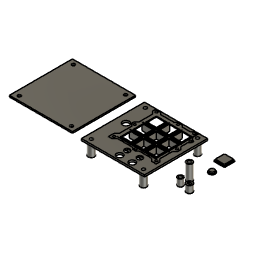
tic_tac_toe (Autodesk Fusion 360 design; units mm, degrees)
Autodesk Fusion 360 part; units mm, degrees
sketch "Sketch1" plane through (0, 0, 0) normal (0, 0, 1) x (1, 0, 0)
  line L0 (0, 0) -> (70, 0)
  line L1 (70, 0) -> (70, 70)
  line L2 (70, 70) -> (0, 70)
  line L3 (0, 70) -> (0, 0)
  circle A0 centre (6, 65) radius 1.75
  circle A1 centre (64, 65) radius 1.75
  circle A2 centre (64, 5) radius 1.75
  circle A3 centre (6, 5) radius 1.75
  line L4 (19, 64.2) -> (32, 64.2)
  line L5 (32, 64.2) -> (32, 51.2)
  line L6 (32, 51.2) -> (19, 51.2)
  line L7 (19, 51.2) -> (19, 64.2)
  line L8 (20, 63.2) -> (31, 63.2)
  line L9 (31, 63.2) -> (31, 52.2)
  line L10 (31, 52.2) -> (20, 52.2)
  line L11 (20, 52.2) -> (20, 63.2)
  line L12 (34, 63.2) -> (45, 63.2)
  line L13 (45, 52.2) -> (34, 52.2)
  line L14 (46, 64.2) -> (46, 51.2)
  line L15 (34, 52.2) -> (34, 63.2)
  line L16 (33, 51.2) -> (33, 64.2)
  line L17 (46, 51.2) -> (33, 51.2)
  line L18 (45, 63.2) -> (45, 52.2)
  line L19 (33, 64.2) -> (46, 64.2)
  line L20 (48, 63.2) -> (59, 63.2)
  line L21 (48, 52.2) -> (48, 63.2)
  line L22 (59, 52.2) -> (48, 52.2)
  line L23 (47, 51.2) -> (47, 64.2)
  line L24 (60, 51.2) -> (47, 51.2)
  line L25 (47, 64.2) -> (60, 64.2)
  line L26 (60, 64.2) -> (60, 51.2)
  line L27 (59, 63.2) -> (59, 52.2)
  line L28 (46, 50.2) -> (46, 37.2)
  line L29 (31, 49.2) -> (31, 38.2)
  line L30 (33, 50.2) -> (46, 50.2)
  line L31 (31, 38.2) -> (20, 38.2)
  line L32 (59, 49.2) -> (59, 38.2)
  line L33 (45, 38.2) -> (34, 38.2)
  line L34 (32, 50.2) -> (32, 37.2)
  line L35 (60, 50.2) -> (60, 37.2)
  line L36 (34, 49.2) -> (45, 49.2)
  line L37 (48, 38.2) -> (48, 49.2)
  line L38 (60, 37.2) -> (47, 37.2)
  line L39 (20, 38.2) -> (20, 49.2)
  line L40 (19, 50.2) -> (32, 50.2)
  line L41 (34, 38.2) -> (34, 49.2)
  line L42 (33, 37.2) -> (33, 50.2)
  line L43 (19, 37.2) -> (19, 50.2)
  line L44 (46, 37.2) -> (33, 37.2)
  line L45 (45, 49.2) -> (45, 38.2)
  line L46 (47, 37.2) -> (47, 50.2)
  line L47 (20, 49.2) -> (31, 49.2)
  line L48 (48, 49.2) -> (59, 49.2)
  line L49 (47, 50.2) -> (60, 50.2)
  line L50 (59, 38.2) -> (48, 38.2)
  line L51 (32, 37.2) -> (19, 37.2)
  line L52 (32, 36.2) -> (32, 23.2)
  line L53 (19, 23.2) -> (19, 36.2)
  line L54 (34, 24.2) -> (34, 35.2)
  line L55 (48, 35.2) -> (59, 35.2)
  line L56 (60, 36.2) -> (60, 23.2)
  line L57 (34, 35.2) -> (45, 35.2)
  line L58 (45, 24.2) -> (34, 24.2)
  line L59 (48, 24.2) -> (48, 35.2)
  line L60 (46, 23.2) -> (33, 23.2)
  line L61 (47, 36.2) -> (60, 36.2)
  line L62 (33, 36.2) -> (46, 36.2)
  line L63 (20, 24.2) -> (20, 35.2)
  line L64 (31, 24.2) -> (20, 24.2)
  line L65 (31, 35.2) -> (31, 24.2)
  line L66 (47, 23.2) -> (47, 36.2)
  line L67 (60, 23.2) -> (47, 23.2)
  line L68 (33, 23.2) -> (33, 36.2)
  line L69 (19, 36.2) -> (32, 36.2)
  line L70 (45, 35.2) -> (45, 24.2)
  line L71 (59, 35.2) -> (59, 24.2)
  line L72 (46, 36.2) -> (46, 23.2)
  line L73 (59, 24.2) -> (48, 24.2)
  line L74 (20, 35.2) -> (31, 35.2)
  line L75 (32, 23.2) -> (19, 23.2)
  circle A4 centre (10, 39.5) radius 3.75
  circle A5 centre (36.9, 14) radius 3
  circle A6 centre (50.9, 14) radius 3
  circle A7 centre (36.9, 14) radius 4
  circle A8 centre (50.9, 14) radius 4
  circle A9 centre (37.25, 5.25) radius 3.5
  circle A10 centre (51.25, 5.25) radius 3.5
  circle A11 centre (16, 67.2) radius 1
  circle A12 centre (58, 67.2) radius 1
  circle A13 centre (16, 43.2) radius 1
  circle A14 centre (16, 20.2) radius 1
  circle A15 centre (63, 20.2) radius 1
  circle A16 centre (63, 43.2) radius 1
  circle A17 centre (40, 20.2) radius 1
  circle A18 centre (40, 67.2) radius 1
  circle A19 centre (63, 58.2) radius 1
  dimension "d1" = 70
  dimension "d2" = 70
  dimension "d3" = 3.5
  dimension "d4" = 6
  dimension "d5" = 5
  dimension "d6" = 3.5
  dimension "d7" = 3.5
  dimension "d8" = 3.5
  dimension "d9" = 6
  dimension "d10" = 5
  dimension "d11" = 6
  dimension "d12" = 5
  dimension "d13" = 5
  dimension "d14" = 6
  dimension "d15" = 13
  dimension "d16" = 13
  dimension "d17" = 19
  dimension "d18" = 5.8
  dimension "d19" = 11
  dimension "d20" = 11
  dimension "d21" = 1
  dimension "d22" = 1
  dimension "d23" = 13
  dimension "d24" = 13
  dimension "d25" = 11
  dimension "d26" = 11
  dimension "d27" = 1
  dimension "d28" = 1
  dimension "d29" = 13
  dimension "d30" = 13
  dimension "d31" = 11
  dimension "d32" = 11
  dimension "d33" = 1
  dimension "d34" = 1
  dimension "d35" = 13
  dimension "d36" = 13
  dimension "d37" = 11
  dimension "d38" = 11
  dimension "d39" = 1
  dimension "d40" = 1
  dimension "d41" = 13
  dimension "d42" = 13
  dimension "d43" = 11
  dimension "d44" = 11
  dimension "d45" = 1
  dimension "d46" = 1
  dimension "d47" = 13
  dimension "d48" = 13
  dimension "d49" = 11
  dimension "d50" = 11
  dimension "d51" = 1
  dimension "d52" = 1
  dimension "d53" = 13
  dimension "d54" = 13
  dimension "d55" = 11
  dimension "d56" = 11
  dimension "d57" = 1
  dimension "d58" = 1
  dimension "d59" = 13
  dimension "d60" = 13
  dimension "d61" = 11
  dimension "d62" = 11
  dimension "d63" = 1
  dimension "d64" = 1
  dimension "d65" = 13
  dimension "d66" = 13
  dimension "d67" = 11
  dimension "d68" = 11
  dimension "d69" = 1
  dimension "d70" = 1
  dimension "d71" = 7.5
  dimension "d72" = 30.5
  dimension "d73" = 10
  dimension "d74" = 6
  dimension "d75" = 14
  dimension "d76" = 36.9
  dimension "d77" = 6
  dimension "d78" = 14
  dimension "d79" = 14
  dimension "d80" = 8
  dimension "d81" = 8
  dimension "d82" = 7
  dimension "d83" = 5.25
  dimension "d84" = 37.25
  dimension "d85" = 7
  dimension "d86" = 14
  dimension "d87" = 5.25
  dimension "d88" = 2
  dimension "d89" = 3
  dimension "d90" = 3
  dimension "d91" = 2
  dimension "d93" = 3
  dimension "d94" = 2
  dimension "d95" = 2
  dimension "d96" = 21
  dimension "d97" = 3
  dimension "d98" = 2
  dimension "d99" = 3
  dimension "d100" = 3
  dimension "d101" = 2
  dimension "d102" = 3
  dimension "d103" = 3
  dimension "d104" = 2
  dimension "d105" = 3
  dimension "d106" = 21
  dimension "d107" = 2
  dimension "d108" = 21
  dimension "d109" = 3
  dimension "d110" = 2
  dimension "d111" = 3
  dimension "d112" = 21
  dimension "d148" = 2
  constraint horizontal L0
  constraint vertical L1
  constraint horizontal L2
  constraint vertical L3
  constraint coincident L0.start L3.end
  constraint horizontal L4
  constraint vertical L5
  constraint horizontal L6
  constraint vertical L7
  constraint horizontal L8
  constraint vertical L9
  constraint horizontal L10
  constraint vertical L11
  constraint horizontal L19
  constraint vertical L14
  constraint horizontal L17
  constraint vertical L16
  constraint horizontal L12
  constraint vertical L18
  constraint horizontal L13
  constraint vertical L15
  constraint horizontal L25
  constraint vertical L26
  constraint horizontal L24
  constraint vertical L23
  constraint horizontal L20
  constraint vertical L27
  constraint horizontal L22
  constraint vertical L21
  constraint horizontal L40
  constraint vertical L34
  constraint horizontal L51
  constraint vertical L43
  constraint horizontal L47
  constraint vertical L29
  constraint horizontal L31
  constraint vertical L39
  constraint horizontal L30
  constraint vertical L28
  constraint horizontal L44
  constraint vertical L42
  constraint horizontal L36
  constraint vertical L45
  constraint horizontal L33
  constraint vertical L41
  constraint horizontal L49
  constraint vertical L35
  constraint horizontal L38
  constraint vertical L46
  constraint horizontal L48
  constraint vertical L32
  constraint horizontal L50
  constraint vertical L37
  constraint horizontal L69
  constraint vertical L52
  constraint horizontal L75
  constraint vertical L53
  constraint horizontal L74
  constraint vertical L65
  constraint horizontal L64
  constraint vertical L63
  constraint horizontal L62
  constraint vertical L72
  constraint horizontal L60
  constraint vertical L68
  constraint horizontal L57
  constraint vertical L70
  constraint horizontal L58
  constraint vertical L54
  constraint horizontal L61
  constraint vertical L56
  constraint horizontal L67
  constraint vertical L66
  constraint horizontal L55
  constraint vertical L71
  constraint horizontal L73
  constraint vertical L59
  constraint concentric A5 A7
  constraint concentric A6 A8
  measures "d1" distance of L0.start L0.end
  measures "d2" distance of L0.start L2.end
  measures "d3" diameter of A0
  measures "d4" distance of L3 A0.centre
  measures "d5" distance of L2 A0.centre
  measures "d6" diameter of A1
  measures "d7" diameter of A2
  measures "d8" diameter of A3
  measures "d9" distance of L1 A1.centre
  measures "d10" distance of L2 A1.centre
  measures "d11" distance of L1 A2.centre
  measures "d12" distance of L0 A2.centre
  measures "d13" distance of L0 A3.centre
  measures "d14" distance of L3 A3.centre
  measures "d15" distance of L4.start L4.end
  measures "d16" distance of L4.start L6.end
  measures "d17" distance of L3 L4.start
  measures "d18" distance of L2 L4
  measures "d19" distance of L8.start L8.end
  measures "d20" distance of L8.start L10.end
  measures "d21" distance of L4 L8
  measures "d22" distance of L7 L11
  measures "d23" distance of L16.end L14.start
  measures "d24" distance of L16.start L16.end
  measures "d25" distance of L12.end L12.start
  measures "d26" distance of L12.start L13.end
  measures "d27" distance of L12 L19
  measures "d28" distance of L15 L16
  measures "d29" distance of L23.end L25.end
  measures "d30" distance of L23.start L23.end
  measures "d31" distance of L20.end L20.start
  measures "d32" distance of L20.start L21.start
  measures "d33" distance of L20 L25
  measures "d34" distance of L21 L23
  measures "d35" distance of L40.start L34.start
  measures "d36" distance of L43.start L40.start
  measures "d37" distance of L29.start L39.end
  measures "d38" distance of L39.end L31.end
  measures "d39" distance of L40 L47
  measures "d40" distance of L39 L43
  measures "d41" distance of L30.start L28.start
  measures "d42" distance of L42.start L30.start
  measures "d43" distance of L36.end L36.start
  measures "d44" distance of L33.end L36.start
  measures "d45" distance of L30 L36
  measures "d46" distance of L41 L42
  measures "d47" distance of L46.end L35.start
  measures "d48" distance of L38.end L46.end
  measures "d49" distance of L37.end L32.start
  measures "d50" distance of L37.start L37.end
  measures "d51" distance of L48 L49
  measures "d52" distance of L37 L46
  measures "d53" distance of L53.end L52.start
  measures "d54" distance of L53.end L53.start
  measures "d55" distance of L65.start L63.end
  measures "d56" distance of L63.start L63.end
  measures "d57" distance of L69 L74
  measures "d58" distance of L53 L63
  measures "d59" distance of L62.end L62.start
  measures "d60" distance of L60.end L62.start
  measures "d61" distance of L57.end L54.end
  measures "d62" distance of L54.start L54.end
  measures "d63" distance of L57 L62
  measures "d64" distance of L54 L68
  measures "d65" distance of L56.start L61.start
  measures "d66" distance of L61.start L66.start
  measures "d67" distance of L55.start L55.end
  measures "d68" distance of L59.start L55.start
  measures "d69" distance of L55 L61
  measures "d70" distance of L59 L66
  measures "d71" diameter of A4
  measures "d72" distance of L2 A4.centre
  measures "d73" distance of L3 A4.centre
  measures "d74" diameter of A5
  measures "d75" distance of L0 A5.centre
  measures "d76" distance of L3 A5.centre
  measures "d77" diameter of A6
  measures "d78" distance of A5.centre A6.centre
  measures "d79" distance of L0 A6.centre
  measures "d80" diameter of A7
  measures "d81" diameter of A8
  measures "d82" diameter of A9
  measures "d83" distance of L0 A9.centre
  measures "d84" distance of L3 A9.centre
  measures "d85" diameter of A10
  measures "d86" horizontal distance of A9.centre A10.centre
  measures "d87" distance of L0 A10.centre
  measures "d88" diameter of A11
  measures "d89" horizontal distance of L4.start A11.centre
  measures "d90" vertical distance of L4.start A11.centre
  measures "d91" diameter of A12
  measures "d93" distance of L25 A12.centre
  measures "d94" distance of L26 A12.centre
  measures "d95" diameter of A13
  measures "d96" distance of L4 A13.centre
  measures "d97" distance of L7 A13.centre
  measures "d98" diameter of A14
  measures "d99" distance of L75 A14.centre
  measures "d100" distance of L53 A14.centre
  measures "d101" diameter of A15
  measures "d102" distance of L56 A15.centre
  measures "d103" distance of L67 A15.centre
  measures "d104" diameter of A16
  measures "d105" distance of L35 A16.centre
  measures "d106" distance of L25 A16.centre
  measures "d107" diameter of A17
  measures "d108" distance of L53 A17.centre
  measures "d109" distance of L60 A17.centre
  measures "d110" diameter of A18
  measures "d111" distance of L19 A18.centre
  measures "d112" distance of L7 A18.centre
  measures "d148" diameter of A19
extrude "Extrude1" add sketch "Sketch1" against normal blind 1 contours L0 L1 L2 L3 | L4 L5 L6 L7 | L14 L16 L17 L19 | L23 L24 L25 L26 | L28 L30 L42 L44 | L34 L40 L43 L51 | L35 L38 L46 L49 | L52 L53 L69 L75 | L56 L61 L66 L67 | L60 L62 L68 L72 | A7 | A8 | A19 makes body 1
extrude "Extrude2" add sketch "Sketch1" against normal blind 2 contours L0 L1 L2 L3 | A19 bodies 1
extrude "Extrude3" add sketch "Sketch1" against normal blind 3 contours A11 | A12 | A13 | A14 | A15 | A16 | A17 | A18 bodies 1
sketch "Sketch2" plane through (0, 0, 0) normal (0, 0, 1) x (1, 0, 0)
  line L0 (14, 69) -> (19, 69)
  line L1 (19, 69) -> (21, 67)
  line L2 (21, 67) -> (36, 67)
  line L3 (36, 67) -> (38, 69)
  line L4 (38, 69) -> (43, 69)
  line L5 (43, 69) -> (45, 67)
  line L6 (45, 67) -> (54, 67)
  line L7 (54, 67) -> (56, 69)
  line L8 (56, 69) -> (60.5, 69)
  line L9 (60.5, 69) -> (60.5, 62.9002)
  line L10 (60.5, 62.9002) -> (63.0154, 60.3847)
  line L11 (63, 52.2579) -> (63, 47.3478)
  line L12 (63, 47.3478) -> (65.8696, 44.4783)
  line L13 (65.8696, 44.4783) -> (65.8696, 40.8696)
  line L14 (65.8696, 40.8696) -> (63, 38)
  line L15 (63, 38) -> (63, 24)
  line L16 (63, 24) -> (66, 21)
  line L17 (66, 21) -> (66, 18)
  line L18 (66, 18) -> (66, 17)
  line L19 (66, 17) -> (61, 17)
  line L20 (61, 17) -> (59, 19)
  line L21 (59, 19) -> (58, 20)
  line L22 (58, 20) -> (44, 20)
  line L23 (44, 20) -> (42, 18)
  line L24 (42, 18) -> (39, 18)
  line L25 (39, 18) -> (37, 20)
  line L26 (37, 20) -> (20, 20)
  line L27 (20, 20) -> (17, 17)
  line L28 (17, 17) -> (13, 17)
  line L29 (13, 17) -> (13, 23)
  line L30 (13, 23) -> (16, 26)
  line L31 (16, 26) -> (16, 40)
  line L32 (16, 40) -> (13, 43)
  line L33 (13, 43) -> (13, 45)
  line L34 (13, 45) -> (16, 48)
  line L35 (16, 48) -> (16, 63)
  line L36 (16, 63) -> (13, 66)
  line L37 (13, 66) -> (13, 69)
  line L38 (13, 69) -> (14, 69)
  line L39 (20, 63.2) -> (31, 63.2)
  line L40 (31, 63.2) -> (31, 63.1885)
  line L41 (31, 63.1885) -> (32.5, 63.1885)
  line L42 (32.5, 63.1885) -> (32.5, 51)
  line L43 (32.5, 51) -> (20.0056, 51)
  line L44 (20.0056, 51) -> (20.0056, 52.2)
  line L45 (20.0056, 52.2) -> (20, 52.2)
  line L46 (20, 52.2) -> (20, 63.2)
  line L47 (34, 52.2) -> (34, 63.2)
  line L48 (46.5, 63.1973) -> (46.5, 51)
  line L49 (46.5, 51) -> (33.9973, 51)
  line L50 (34, 63.2) -> (45, 63.2)
  line L51 (33.9973, 51) -> (33.9973, 52.2)
  line L52 (45, 63.2) -> (45, 63.1973)
  line L53 (33.9973, 52.2) -> (34, 52.2)
  line L54 (45, 63.1973) -> (46.5, 63.1973)
  line L55 (47.9901, 51) -> (47.9901, 52.2)
  line L56 (60.5, 63.178) -> (60.5, 51)
  line L57 (60.5, 51) -> (47.9901, 51)
  line L58 (59, 63.178) -> (60.5, 63.178)
  line L59 (48, 63.2) -> (59, 63.2)
  line L60 (59, 63.2) -> (59, 63.178)
  line L61 (48, 52.2) -> (48, 63.2)
  line L62 (47.9901, 52.2) -> (48, 52.2)
  line L63 (34, 49.2) -> (45, 49.2)
  line L64 (33.9963, 38.2) -> (34, 38.2)
  line L65 (47.987, 37) -> (47.987, 38.2)
  line L66 (48, 49.2) -> (59, 49.2)
  line L67 (20, 49.2) -> (31, 49.2)
  line L68 (60.5, 49.1894) -> (60.5, 37)
  line L69 (47.987, 38.2) -> (48, 38.2)
  line L70 (31, 49.1925) -> (32.5, 49.1925)
  line L71 (32.5, 49.1925) -> (32.5, 37)
  line L72 (45, 49.1919) -> (46.5, 49.1919)
  line L73 (31, 49.2) -> (31, 49.1925)
  line L74 (46.5, 37) -> (33.9963, 37)
  line L75 (48, 38.2) -> (48, 49.2)
  line L76 (59, 49.1894) -> (60.5, 49.1894)
  line L77 (19.9937, 37) -> (19.9937, 38.2)
  line L78 (32.5, 37) -> (19.9937, 37)
  line L79 (59, 49.2) -> (59, 49.1894)
  line L80 (34, 38.2) -> (34, 49.2)
  line L81 (60.5, 37) -> (47.987, 37)
  line L82 (19.9937, 38.2) -> (20, 38.2)
  line L83 (45, 49.2) -> (45, 49.1919)
  line L84 (33.9963, 37) -> (33.9963, 38.2)
  line L85 (20, 38.2) -> (20, 49.2)
  line L86 (46.5, 49.1919) -> (46.5, 37)
  line L87 (59, 35.197) -> (60.5, 35.197)
  line L88 (20, 35.2) -> (31, 35.2)
  line L89 (19.9925, 24.2) -> (20, 24.2)
  line L90 (33.998, 24.2) -> (34, 24.2)
  line L91 (34, 35.2) -> (45, 35.2)
  line L92 (48, 35.2) -> (59, 35.2)
  line L93 (31, 35.1568) -> (32.5, 35.1568)
  line L94 (32.5, 35.1568) -> (32.5, 23)
  line L95 (45, 35.2) -> (45, 35.196)
  line L96 (46.5, 35.196) -> (46.5, 23)
  line L97 (48, 24.2) -> (48, 35.2)
  line L98 (59, 35.2) -> (59, 35.197)
  line L99 (32.5, 23) -> (19.9925, 23)
  line L100 (46.5, 23) -> (33.998, 23)
  line L101 (47.9985, 23) -> (47.9985, 24.2)
  line L102 (19.9925, 23) -> (19.9925, 24.2)
  line L103 (33.998, 23) -> (33.998, 24.2)
  line L104 (60.5, 35.197) -> (60.5, 23)
  line L105 (34, 24.2) -> (34, 35.2)
  line L106 (31, 35.2) -> (31, 35.1568)
  line L107 (20, 24.2) -> (20, 35.2)
  line L108 (47.9985, 24.2) -> (48, 24.2)
  line L109 (60.5, 23) -> (47.9985, 23)
  line L110 (45, 35.196) -> (46.5, 35.196)
  circle A0 centre (63, 43.2) radius 1.3
  circle A1 centre (58, 67.2) radius 1.3
  circle A2 centre (40, 67.2) radius 1.3
  circle A3 centre (16, 67.2) radius 1.3
  circle A4 centre (16, 43.2) radius 1.3
  circle A5 centre (16, 20.2) radius 1.3
  circle A6 centre (40, 20.2) radius 1.3
  circle A7 centre (63, 20.2) radius 1.3
  circle A8 centre (63, 58.2) radius 1.3
  line L111 (62.9593, 60.4409) -> (65.2008, 59.4959)
  line L112 (63, 52.2579) -> (63, 55)
  line L113 (63, 55) -> (65.2, 57.4)
  line L114 (65.2, 57.4) -> (65.2008, 59.4959)
  point P0 (60.5, 46)
  point P1 (60.5, 32)
  dimension "d119" = 2.6
  dimension "d120" = 2.6
  dimension "d121" = 2.6
  dimension "d122" = 2.6
  dimension "d123" = 2.6
  dimension "d124" = 2.6
  dimension "d125" = 2.6
  dimension "d126" = 2.6
  dimension "d145" = 2.6
  constraint horizontal L0
  constraint horizontal L2
  constraint perpendicular L1 L3
  constraint parallel L2 L4
  constraint perpendicular L3 L5
  constraint parallel L4 L6
  constraint perpendicular L5 L7
  constraint parallel L6 L8
  constraint perpendicular L8 L9
  constraint perpendicular L7 L10
  constraint perpendicular L8 L11
  constraint parallel L10 L12
  constraint parallel L11 L13
  constraint perpendicular L12 L14
  constraint parallel L13 L15
  constraint perpendicular L14 L16
  constraint parallel L15 L17
  constraint parallel L17 L18
  constraint perpendicular L17 L19
  constraint parallel L16 L20
  constraint parallel L20 L21
  constraint parallel L19 L22
  constraint perpendicular L21 L23
  constraint parallel L22 L24
  constraint parallel L21 L25
  constraint parallel L24 L26
  constraint perpendicular L25 L27
  constraint parallel L26 L28
  constraint perpendicular L28 L29
  constraint perpendicular L25 L30
  constraint perpendicular L28 L31
  constraint perpendicular L30 L32
  constraint parallel L31 L33
  constraint perpendicular L32 L34
  constraint parallel L33 L35
  constraint perpendicular L34 L36
  constraint parallel L35 L37
  constraint perpendicular L37 L38
  constraint perpendicular L37 L39
  constraint perpendicular L39 L40
  constraint perpendicular L40 L41
  constraint perpendicular L41 L42
  constraint perpendicular L42 L43
  constraint perpendicular L43 L44
  constraint perpendicular L44 L45
  constraint perpendicular L50 L52
  constraint perpendicular L52 L54
  constraint perpendicular L48 L54
  constraint perpendicular L48 L49
  constraint perpendicular L49 L51
  constraint perpendicular L51 L53
  constraint perpendicular L59 L60
  constraint perpendicular L58 L60
  constraint perpendicular L56 L58
  constraint perpendicular L56 L57
  constraint perpendicular L55 L57
  constraint perpendicular L55 L62
  constraint perpendicular L67 L73
  constraint perpendicular L70 L73
  constraint perpendicular L70 L71
  constraint perpendicular L71 L78
  constraint perpendicular L77 L78
  constraint perpendicular L77 L82
  constraint perpendicular L63 L83
  constraint perpendicular L72 L83
  constraint perpendicular L72 L86
  constraint perpendicular L74 L86
  constraint perpendicular L74 L84
  constraint perpendicular L64 L84
  constraint perpendicular L66 L79
  constraint perpendicular L76 L79
  constraint perpendicular L68 L76
  constraint perpendicular L68 L81
  constraint perpendicular L65 L81
  constraint perpendicular L65 L69
  constraint perpendicular L88 L106
  constraint perpendicular L93 L106
  constraint perpendicular L93 L94
  constraint perpendicular L94 L99
  constraint perpendicular L99 L102
  constraint perpendicular L89 L102
  constraint perpendicular L91 L95
  constraint perpendicular L95 L110
  constraint perpendicular L96 L110
  constraint perpendicular L96 L100
  constraint perpendicular L100 L103
  constraint perpendicular L90 L103
  constraint perpendicular L92 L98
  constraint perpendicular L87 L98
  constraint perpendicular L87 L104
  constraint perpendicular L104 L109
  constraint perpendicular L101 L109
  constraint perpendicular L101 L108
  constraint coincident L10 L111.start
  constraint parallel L11 L112
  measures "d119" diameter of A3
  measures "d120" diameter of A1
  measures "d121" diameter of A4
  measures "d122" diameter of A5
  measures "d123" diameter of A7
  measures "d124" diameter of A0
  measures "d125" diameter of A6
  measures "d126" diameter of A2
  measures "d145" diameter of A8
extrude "Extrude4" add sketch "Sketch2" against normal blind 0.6 separate body contours L0 L1 L2 L3 L4 L5 L6 L7 L8 L9 L10 L11 L12 L13 L14 L15 L16 L17 L18 L19 L20 L21 L22 L23 L24 L25 L26 L27 L28 L29 L30 L31 L32 L33 L34 L35 L36 L37 L38 L55 L56 L57 L58 L59 L60 L61 L62 L111 L112 L113 L114 | A8 makes body 2
sketch "Sketch3" plane through (0, 0, 0) normal (0, 0, 1) x (-1, 0, 0)
  circle A0 centre (-40, -20.2) radius 1.3
  circle A1 centre (-40, -67.2) radius 1.3
  circle A2 centre (-58, -67.2) radius 1.3
  line L0 (-19.9925, -24.2) -> (-20, -24.2)
  line L1 (-20, -24.2) -> (-20, -35.2)
  line L2 (-20, -35.2) -> (-31, -35.2)
  line L3 (-31, -35.2) -> (-31, -35.1568)
  line L4 (-31, -35.1568) -> (-32.5, -35.1568)
  line L5 (-32.5, -35.1568) -> (-32.5, -23)
  line L6 (-32.5, -23) -> (-19.9925, -23)
  line L7 (-19.9925, -23) -> (-19.9925, -24.2)
  line L8 (-47.9901, -51) -> (-47.9901, -52.2)
  line L9 (-47.9901, -52.2) -> (-48, -52.2)
  line L10 (-48, -52.2) -> (-48, -63.2)
  line L11 (-48, -63.2) -> (-59, -63.2)
  line L12 (-59, -63.2) -> (-59, -63.178)
  line L13 (-59, -63.178) -> (-60.5, -63.178)
  line L14 (-60.5, -62.9002) -> (-60.5, -51)
  line L15 (-60.5, -51) -> (-47.9901, -51)
  circle A3 centre (-63, -43.2) radius 1.3
  circle A4 centre (-63, -20.2) radius 1.3
  line L16 (-19.9937, -38.2) -> (-20, -38.2)
  line L17 (-20, -38.2) -> (-20, -49.2)
  line L18 (-20, -49.2) -> (-31, -49.2)
  line L19 (-31, -49.2) -> (-31, -49.1925)
  line L20 (-31, -49.1925) -> (-32.5, -49.1925)
  line L21 (-32.5, -49.1925) -> (-32.5, -37)
  line L22 (-32.5, -37) -> (-19.9937, -37)
  line L23 (-19.9937, -37) -> (-19.9937, -38.2)
  line L24 (-45, -63.2) -> (-45, -63.1973)
  line L25 (-45, -63.1973) -> (-46.5, -63.1973)
  line L26 (-46.5, -63.1973) -> (-46.5, -51)
  line L27 (-46.5, -51) -> (-33.9973, -51)
  line L28 (-33.9973, -51) -> (-33.9973, -52.2)
  line L29 (-33.9973, -52.2) -> (-34, -52.2)
  line L30 (-34, -52.2) -> (-34, -63.2)
  line L31 (-34, -63.2) -> (-45, -63.2)
  circle A5 centre (-16, -43.2) radius 1.3
  line L32 (-60.5, -49.1894) -> (-60.5, -37)
  line L33 (-60.5, -37) -> (-47.987, -37)
  line L34 (-47.987, -37) -> (-47.987, -38.2)
  line L35 (-47.987, -38.2) -> (-48, -38.2)
  line L36 (-48, -38.2) -> (-48, -49.2)
  line L37 (-48, -49.2) -> (-59, -49.2)
  line L38 (-59, -49.2) -> (-59, -49.1894)
  line L39 (-59, -49.1894) -> (-60.5, -49.1894)
  circle A6 centre (-16, -67.2) radius 1.3
  line L40 (-20.0056, -52.2) -> (-20, -52.2)
  line L41 (-20, -52.2) -> (-20, -63.2)
  line L42 (-20, -63.2) -> (-31, -63.2)
  line L43 (-31, -63.2) -> (-31, -63.1885)
  line L44 (-31, -63.1885) -> (-32.5, -63.1885)
  line L45 (-32.5, -63.1885) -> (-32.5, -51)
  line L46 (-32.5, -51) -> (-20.0056, -51)
  line L47 (-20.0056, -51) -> (-20.0056, -52.2)
  line L48 (-60.5, -35.197) -> (-60.5, -23)
  line L49 (-60.5, -23) -> (-47.9985, -23)
  line L50 (-47.9985, -23) -> (-47.9985, -24.2)
  line L51 (-47.9985, -24.2) -> (-48, -24.2)
  line L52 (-48, -24.2) -> (-48, -35.2)
  line L53 (-48, -35.2) -> (-59, -35.2)
  line L54 (-59, -35.2) -> (-59, -35.197)
  line L55 (-59, -35.197) -> (-60.5, -35.197)
  circle A7 centre (-16, -20.2) radius 1.3
  line L56 (-45, -49.1919) -> (-46.5, -49.1919)
  line L57 (-46.5, -49.1919) -> (-46.5, -37)
  line L58 (-46.5, -37) -> (-33.9963, -37)
  line L59 (-33.9963, -37) -> (-33.9963, -38.2)
  line L60 (-33.9963, -38.2) -> (-34, -38.2)
  line L61 (-34, -38.2) -> (-34, -49.2)
  line L62 (-34, -49.2) -> (-45, -49.2)
  line L63 (-45, -49.2) -> (-45, -49.1919)
  line L64 (-45, -35.2) -> (-45, -35.196)
  line L65 (-45, -35.196) -> (-46.5, -35.196)
  line L66 (-46.5, -35.196) -> (-46.5, -23)
  line L67 (-46.5, -23) -> (-33.998, -23)
  line L68 (-33.998, -23) -> (-33.998, -24.2)
  line L69 (-33.998, -24.2) -> (-34, -24.2)
  line L70 (-34, -24.2) -> (-34, -35.2)
  line L71 (-34, -35.2) -> (-45, -35.2)
  line L72 (-13, -69) -> (-13, -66)
  line L73 (-13, -66) -> (-16, -63)
  line L74 (-16, -63) -> (-16, -48)
  line L75 (-16, -48) -> (-13, -45)
  line L76 (-13, -45) -> (-13, -43)
  line L77 (-13, -43) -> (-16, -40)
  line L78 (-16, -40) -> (-16, -26)
  line L79 (-16, -26) -> (-13, -23)
  line L80 (-13, -23) -> (-13, -17)
  line L81 (-13, -17) -> (-17, -17)
  line L82 (-17, -17) -> (-20, -20)
  line L83 (-20, -20) -> (-37, -20)
  line L84 (-37, -20) -> (-39, -18)
  line L85 (-39, -18) -> (-42, -18)
  line L86 (-42, -18) -> (-44, -20)
  line L87 (-44, -20) -> (-58, -20)
  line L88 (-58, -20) -> (-61, -17)
  line L89 (-61, -17) -> (-66, -17)
  line L90 (-66, -17) -> (-66, -21)
  line L91 (-66, -21) -> (-63, -24)
  line L92 (-63, -24) -> (-63, -38)
  line L93 (-63, -38) -> (-65.8696, -40.8696)
  line L94 (-65.8696, -40.8696) -> (-65.8696, -44.4783)
  line L95 (-65.8696, -44.4783) -> (-63, -47.3478)
  line L96 (-63, -47.3478) -> (-63, -52.2579)
  line L97 (-62.9593, -60.4409) -> (-60.5, -62.9002)
  line L98 (-60.5, -63.178) -> (-60.5, -69)
  line L99 (-60.5, -69) -> (-56, -69)
  line L100 (-56, -69) -> (-54, -67)
  line L101 (-54, -67) -> (-45, -67)
  line L102 (-45, -67) -> (-43, -69)
  line L103 (-43, -69) -> (-38, -69)
  line L104 (-38, -69) -> (-36, -67)
  line L105 (-36, -67) -> (-21, -67)
  line L106 (-21, -67) -> (-19, -69)
  line L107 (-19, -69) -> (-13, -69)
  line L108 (-17.5, -50.5) -> (-61, -50.5)
  line L109 (-61, -50.5) -> (-61, -49.7)
  line L110 (-61, -49.7) -> (-17.5, -49.7)
  line L111 (-17.5, -49.7) -> (-17.5, -50.5)
  line L112 (-32.7, -64.5) -> (-33.5, -64.5)
  line L113 (-33.5, -64.5) -> (-33.5, -21.74)
  line L114 (-33.5, -21.74) -> (-32.7, -21.74)
  line L115 (-32.7, -21.74) -> (-32.7, -64.5)
  line L116 (-46.7, -64.5) -> (-47.5, -64.5)
  line L117 (-47.5, -64.5) -> (-47.5, -21.722)
  line L118 (-47.5, -21.722) -> (-46.7, -21.722)
  line L119 (-46.7, -21.722) -> (-46.7, -64.5)
  line L120 (-17.5, -36.5) -> (-61.5, -36.5)
  line L121 (-61.5, -36.5) -> (-61.5, -35.7)
  line L122 (-61.5, -35.7) -> (-17.5, -35.7)
  line L123 (-17.5, -35.7) -> (-17.5, -36.5)
  line L124 (-65.2008, -59.4959) -> (-62.9593, -60.4409)
  line L125 (-63, -52.2579) -> (-63, -55)
  line L126 (-63, -55) -> (-65.2, -57.4)
  line L127 (-65.2, -57.4) -> (-65.2008, -59.4959)
  line L128 (-61.4351, -22.5) -> (-17.296, -22.5)
  line L129 (-17.296, -22.5) -> (-17.296, -21.7)
  line L130 (-17.296, -21.7) -> (-61.4351, -21.7)
  line L131 (-61.4351, -21.7) -> (-61.4351, -22.5)
  dimension "d170" = 0.8
  dimension "d171" = 0.8
  dimension "d172" = 0.8
  dimension "d173" = 0.8
  dimension "d174" = 0.8
  constraint horizontal L108
  constraint vertical L109
  constraint horizontal L110
  constraint vertical L111
  constraint horizontal L112
  constraint vertical L113
  constraint horizontal L114
  constraint vertical L115
  constraint horizontal L116
  constraint vertical L117
  constraint horizontal L118
  constraint vertical L119
  constraint horizontal L120
  constraint vertical L121
  constraint horizontal L122
  constraint vertical L123
  constraint horizontal L128
  constraint vertical L129
  constraint horizontal L130
  constraint vertical L131
  measures "d170" distance of L120 L122
  measures "d171" distance of L117 L119
  measures "d172" distance of L113 L115
  measures "d173" distance of L108 L110
  measures "d174" distance of L128 L130
extrude "Extrude5" add sketch "Sketch3" against normal blind 3.5 contours L108 L110 L111 L115 | L108 L112 L113 L115 | L108 L110 L113 L115 | L108 L110 L113 L119 | L110 L113 L115 L120 | L108 L116 L117 L119 | L108 L110 L117 L119 | L113 L115 L120 L122 | L108 L109 L110 L117 | L110 L117 L119 L120 | L113 L119 L120 L122 | L113 L115 L122 L128 | L117 L119 L120 L122 | L113 L114 L115 L128 | L117 L120 L121 L122 | L117 L119 L122 L128 | L117 L118 L119 L128 bodies 2
sketch "Sketch4" plane through (0, 0, 0) normal (0, 0, 1) x (1, 0, 0)
  line L0 (107.6, 62.4) -> (107.6, 52.2)
  line L1 (96.4, 53) -> (96.4, 61.6)
  line L2 (97.2, 62.4) -> (105.8, 62.4)
  line L3 (105.8, 52.2) -> (97.2, 52.2)
  line L4 (106.6, 61.6) -> (106.6, 53)
  line L5 (96.4, 63.4) -> (106.6, 63.4)
  line L6 (95.4, 52.2) -> (95.4, 62.4)
  line L7 (106.6, 51.2) -> (96.4, 51.2)
  arc A0 (96.4, 63.4) -> (95.4, 62.4) centre (96.4, 62.4) ccw
  arc A1 (107.6, 62.4) -> (106.6, 63.4) centre (106.6, 62.4) ccw
  arc A2 (106.6, 51.2) -> (107.6, 52.2) centre (106.6, 52.2) ccw
  arc A3 (95.4, 52.2) -> (96.4, 51.2) centre (96.4, 52.2) ccw
  arc A4 (97.2, 62.4) -> (96.4, 61.6) centre (97.2, 61.6) ccw
  arc A5 (106.6, 61.6) -> (105.8, 62.4) centre (105.8, 61.6) ccw
  arc A6 (105.8, 52.2) -> (106.6, 53) centre (105.8, 53) ccw
  arc A7 (96.4, 53) -> (97.2, 52.2) centre (97.2, 53) ccw
  point P0 (106.6, 62.4)
  point P1 (96.4, 62.4)
  point P2 (96.4, 52.2)
  point P3 (95.4, 51.2)
  point P4 (95.4, 63.4)
  point P5 (107.6, 63.4)
  dimension "d131" = 12.2
  dimension "d132" = 12.2
  dimension "d133" = 10.2
  dimension "d134" = 10.2
  dimension "d135" = 1
  dimension "d136" = 1
  dimension "d151" = 1
  dimension "d152" = 1
  dimension "d153" = 1
  dimension "d154" = 1
  dimension "d155" = 0.8
  dimension "d156" = 0.8
  dimension "d157" = 0.8
  dimension "d158" = 0.8
  constraint horizontal L5
  constraint vertical L0
  constraint horizontal L7
  constraint vertical L6
  constraint horizontal L2
  constraint vertical L4
  constraint horizontal L3
  constraint vertical L1
  constraint coincident P4 L6
  constraint coincident P4 L5
  constraint tangent L6 A0
  constraint tangent L5 A0
  constraint coincident P5 L5
  constraint coincident P5 L0
  constraint tangent L5 A1
  constraint tangent L0 A1
  constraint tangent L7 A2
  constraint tangent L0 A2
  constraint coincident P3 L6
  constraint coincident P3 L7
  constraint tangent L6 A3
  constraint tangent L7 A3
  constraint coincident P1 L1
  constraint coincident P1 L2
  constraint tangent L1 A4
  constraint tangent L2 A4
  constraint coincident P0 L2
  constraint coincident P0 L4
  constraint tangent L2 A5
  constraint tangent L4 A5
  constraint tangent L3 A6
  constraint tangent L4 A6
  constraint coincident P2 L1
  constraint coincident P2 L3
  constraint tangent L1 A7
  constraint tangent L3 A7
  measures "d131" distance of P4 P5
  measures "d132" distance of P3 P4
  measures "d133" distance of P0 A0.centre
  measures "d134" distance of P1 A3.centre
  measures "d135" distance of L2 L5
  measures "d136" distance of L1 L6
  measures "d151" radius of A0
  measures "d152" radius of A1
  measures "d153" radius of A2
  measures "d154" radius of A3
  measures "d155" radius of A4
  measures "d156" radius of A5
  measures "d157" radius of A6
  measures "d158" radius of A7
extrude "Extrude6" add sketch "Sketch4" along normal blind 1.5 separate body contours L1 L2 L3 L4 A4 A5 A6 A7 makes body 3
extrude "Extrude7" add sketch "Sketch4" along normal blind 0.8 bodies 3
extrude "Extrude8" add 1 faces at (100.0667, 55.6, 1.5) along direction (0, 0, 1) blind 0.8 on bodies 3 bodies 3
extrude "Extrude9" add 1 faces at (32.9667, 35.7133, -3.5) along direction (0, 0, -1) blind 5 on bodies 2 bodies 2
extrude "Extrude10" cut sketch "Sketch2" against normal blind 1 contours A8 bodies 2
extrude "Extrude11" add sketch "Sketch1" against normal blind 3 contours A19 bodies 1
extrude "Extrude12" cut sketch "Sketch4" along normal blind 0.3 contours L0 L5 L6 L7 A0 A1 A2 A3 | L1 L2 L3 L4 A4 A5 A6 A7 bodies 3
sketch "Sketch5" plane through (0, 0, -2) normal (0, 0, -1) x (1, 0, 0)
  circle A0 centre (63, -58.2) radius 1
  circle A1 centre (6, -65) radius 1.75
  circle A2 centre (64, -5) radius 1.75
  circle A3 centre (64, -65) radius 1.75
  circle A4 centre (6, -5) radius 1.75
  line L0 (19, -51.2) -> (32, -51.2)
  line L1 (32, -51.2) -> (32, -64.2)
  line L2 (32, -64.2) -> (19, -64.2)
  line L3 (19, -64.2) -> (19, -51.2)
  line L4 (33, -64.2) -> (33, -51.2)
  line L5 (33, -51.2) -> (46, -51.2)
  line L6 (46, -51.2) -> (46, -64.2)
  line L7 (46, -64.2) -> (33, -64.2)
  line L8 (60, -64.2) -> (47, -64.2)
  line L9 (47, -64.2) -> (47, -51.2)
  line L10 (47, -51.2) -> (60, -51.2)
  line L11 (60, -51.2) -> (60, -64.2)
  line L12 (46, -37.2) -> (46, -50.2)
  line L13 (46, -50.2) -> (33, -50.2)
  line L14 (33, -50.2) -> (33, -37.2)
  line L15 (33, -37.2) -> (46, -37.2)
  line L16 (47, -50.2) -> (47, -37.2)
  line L17 (47, -37.2) -> (60, -37.2)
  line L18 (60, -37.2) -> (60, -50.2)
  line L19 (60, -50.2) -> (47, -50.2)
  circle A5 centre (36.9, -14) radius 4
  line L20 (32, -37.2) -> (32, -50.2)
  line L21 (32, -50.2) -> (19, -50.2)
  line L22 (19, -50.2) -> (19, -37.2)
  line L23 (19, -37.2) -> (32, -37.2)
  line L24 (60, -23.2) -> (60, -36.2)
  line L25 (60, -36.2) -> (47, -36.2)
  line L26 (47, -36.2) -> (47, -23.2)
  line L27 (47, -23.2) -> (60, -23.2)
  line L28 (46, -36.2) -> (33, -36.2)
  line L29 (33, -36.2) -> (33, -23.2)
  line L30 (33, -23.2) -> (46, -23.2)
  line L31 (46, -23.2) -> (46, -36.2)
  line L32 (32, -23.2) -> (32, -36.2)
  line L33 (32, -36.2) -> (19, -36.2)
  line L34 (19, -36.2) -> (19, -23.2)
  line L35 (19, -23.2) -> (32, -23.2)
  circle A6 centre (50.9, -14) radius 4
  circle A7 centre (10, -39.5) radius 3.75
  circle A8 centre (37.25, -5.25) radius 3.5
  circle A9 centre (51.25, -5.25) radius 3.5
  circle A10 centre (16, -67.2) radius 1
  circle A11 centre (58, -67.2) radius 1
  circle A12 centre (16, -43.2) radius 1
  circle A13 centre (16, -20.2) radius 1
  circle A14 centre (63, -20.2) radius 1
  circle A15 centre (63, -43.2) radius 1
  circle A16 centre (40, -20.2) radius 1
  circle A17 centre (40, -67.2) radius 1
  line L36 (0, 0) -> (0, -70)
  line L37 (0, -70) -> (70, -70)
  line L38 (70, -70) -> (70, 0)
  line L39 (70, 0) -> (0, 0)
  circle A18 centre (64, -65) radius 3.25
  circle A19 centre (64, -65) radius 1.75
  circle A20 centre (6, -65) radius 3.5
  circle A21 centre (6, -65) radius 1.75
  circle A22 centre (6, -5) radius 3.5
  circle A23 centre (6, -5) radius 1.75
  circle A24 centre (64, -5) radius 3.5
  circle A25 centre (64, -5) radius 1.75
  dimension "d161" = 6.5
  dimension "d162" = 3.5
  dimension "d163" = 7
  dimension "d164" = 7
  dimension "d165" = 7
  constraint concentric A3 A18
  constraint concentric A18 A19
  constraint concentric A1 A20
  constraint concentric A20 A21
  constraint concentric A4 A22
  constraint concentric A22 A23
  constraint concentric A2 A24
  constraint concentric A24 A25
  measures "d161" diameter of A18
  measures "d162" diameter of A19
  measures "d163" diameter of A20
  measures "d164" diameter of A22
  measures "d165" diameter of A24
extrude "Extrude13" add sketch "Sketch5" along normal blind 13.5 contours A18 | A20 | A22 | A24 bodies 1
extrude "Extrude14" add sketch "Sketch3" against normal blind 8.5 contours L113 L114 L115 L117 L118 L119 L128 L129 L130 L131 bodies 2
extrude "Extrude15" add sketch "Sketch3" against normal blind 8.5 contours L115 L120 L122 L123 bodies 2
sketch "Sketch6" plane through (0, 0, 0) normal (0, 0, 1) x (1, 0, 0)
  circle A0 centre (100, 20) radius 3.25
  circle A1 centre (100, 20) radius 1.75
  circle A2 centre (100, 10) radius 3
  circle A3 centre (100, 10) radius 1.75
  dimension "d177" = 6.5
  dimension "d178" = 3.5
  dimension "d181" = 6
  dimension "d182" = 3.5
  constraint concentric A0 A1
  constraint concentric A2 A3
  measures "d177" diameter of A0
  measures "d178" diameter of A1
  measures "d181" diameter of A2
  measures "d182" diameter of A3
extrude "Extrude16" add sketch "Sketch6" along normal blind 17.5 separate body contours A0 makes body 4
extrude "Extrude17" add sketch "Sketch6" along normal blind 8 separate body contours A2 | A3 makes body 5
sketch "Sketch7" plane through (0, 0, 8) normal (0, 0, 1) x (-1, 0, 0)
  circle A0 centre (-100, -10) radius 3
  circle A1 centre (-100, -10) radius 1.75
  dimension "d185" = 3.5
  constraint concentric A0 A1
  measures "d185" diameter of A1
extrude "Extrude18" cut sketch "Sketch7" against normal blind 4 contours A1 bodies 5
fillet "Fillet1" radius 0.5 1 edges at (97.203, 8.9152, 0) on bodies 5
sketch "Sketch8" plane through (0, 0, 0) normal (0, 0, 1) x (1, 0, 0)
  circle A0 centre (110, 10) radius 3.4
  dimension "d190" = 6.8
  measures "d190" diameter of A0
extrude "Extrude19" add sketch "Sketch8" along normal blind 7 separate body makes body 6
sketch "Sketch9" plane through (0, 0, 7) normal (0, 0, 1) x (-1, 0, 0)
  circle A0 centre (-110, -10) radius 3.4
  line L0 (-108.3, -11.2) -> (-111.7, -11.2)
  line L1 (-111.7, -11.2) -> (-111.7, -8.8)
  line L2 (-111.7, -8.8) -> (-108.3, -8.8)
  line L3 (-108.3, -8.8) -> (-108.3, -11.2)
  dimension "d193" = 1.7
  dimension "d194" = 1.7
  dimension "d195" = 1.2
  dimension "d196" = 1.2
  constraint horizontal L0
  constraint vertical L1
  constraint horizontal L2
  constraint vertical L3
  measures "d193" distance of A0.centre L1
  measures "d194" distance of A0.centre L3
  measures "d195" vertical distance of A0.centre L0.end
  measures "d196" distance of A0.centre L2
extrude "Extrude20" add 1 faces at (108.7342, 9.4367, 0) along direction (0, 0, -1) blind 1 on bodies 6 bodies 6
extrude "Extrude21" cut sketch "Sketch9" against normal blind 2.5 contours L0 L1 L2 L3 bodies 6
chamfer "Chamfer1" distance 0.5 angle 45 1 edges at (106.8301, 11.2295, -1) on bodies 6
sketch "Sketch10" plane through (0, 0, 0) normal (0, 0, 1) x (1, 0, 0)
  circle A0 centre (105, 40) radius 3.5
  circle A1 centre (105, 40) radius 2.6
  dimension "d202" = 7
  dimension "d203" = 5.2
  constraint concentric A0 A1
  measures "d202" diameter of A0
  measures "d203" diameter of A1
extrude "Extrude22" add sketch "Sketch10" along normal blind 2 separate body contours A1 makes body 7
extrude "Extrude23" add sketch "Sketch10" along normal blind 0.5 bodies 7
sketch "Sketch11" plane through (0, 0, 0) normal (0, 0, 1) x (1, 0, 0)
  line L0 (-80, 70) -> (-80, 0)
  line L1 (-10, 70) -> (-80, 70)
  line L2 (-10, 0) -> (-10, 70)
  line L3 (-80, 0) -> (-10, 0)
  circle A0 centre (-74, 65) radius 1.75
  circle A1 centre (-16, 65) radius 1.75
  circle A2 centre (-16, 5) radius 1.75
  circle A3 centre (-74, 5) radius 1.75
  dimension "d208" = 70
  dimension "d209" = 70
  dimension "d210" = 3.5
  dimension "d211" = 6
  dimension "d212" = 5
  dimension "d213" = 3.5
  dimension "d214" = 3.5
  dimension "d215" = 3.5
  dimension "d216" = 6
  dimension "d217" = 5
  dimension "d218" = 6
  dimension "d219" = 5
  dimension "d220" = 5
  dimension "d221" = 6
  constraint horizontal L3
  constraint vertical L2
  constraint horizontal L1
  constraint vertical L0
  measures "d208" distance of L0.end L2.start
  measures "d209" distance of L0.end L0.start
  measures "d210" diameter of A0
  measures "d211" distance of A0.centre L0
  measures "d212" distance of A0.centre L1
  measures "d213" diameter of A1
  measures "d214" diameter of A2
  measures "d215" diameter of A3
  measures "d216" distance of A1.centre L2
  measures "d217" distance of A1.centre L1
  measures "d218" distance of A2.centre L2
  measures "d219" distance of A2.centre L3
  measures "d220" distance of A3.centre L3
  measures "d221" distance of A3.centre L0
extrude "Extrude24" add sketch "Sketch11" along normal blind 1.6 separate body makes body 8
